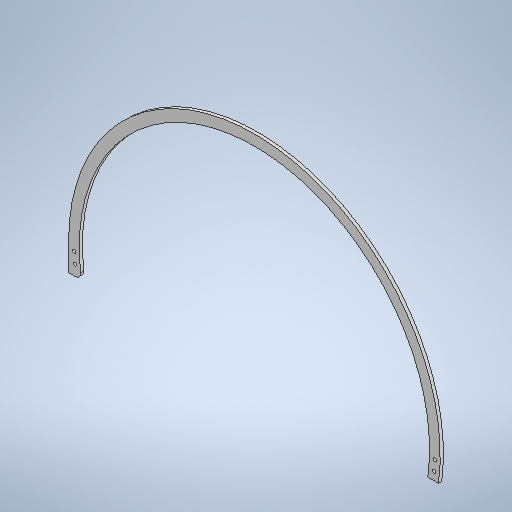
# Autodesk Inventor part: light_ball_space_out
Saved by Autodesk Inventor 2025.1 (Build 291241000, 241)
## iProperties
Created: 2025-05-06
Part Number: light_ball_space_out
Material: 一般
Document SubType Name: Modeling
Designer: yuki0520
Density: 1 g/cm^3
Appearance: 既定
Author: yuki0520
Autodesk Inventor part; units mm, degrees
ref_plane "YZ Plane" through (0, 0, 0) normal (1, 0, 0) x (0, 1, 0)
ref_plane "XZ Plane" through (0, 0, 0) normal (0, 1, 0) x (-1, 0, 0)
ref_plane "XY Plane" through (0, 0, 0) normal (0, 0, 1) x (1, 0, 0)
sketch "スケッチ1" plane through (0, 0, 0) normal (0, 0, 1) x (1, 0, 0)
  line L0 (195, -7.5) -> (-195, -7.5)
  line L1 (-195, -7.5) -> (-195, 7.5)
  line L2 (-195, 7.5) -> (195, 7.5)
  line L3 (195, 7.5) -> (195, -7.5)
  line L4 (195, -7.5) -> (-195, 7.5) construction
  line L5 (-195, -7.5) -> (195, 7.5) construction
  circle A0 centre (0, 70.8153) radius 120
  line L6 (0, -7.5) -> (0, 7.5)
  circle A1 centre (-127.5, -22.5) radius 38
  line L7 (-175, -5) -> (-135, -5)
  line L8 (-135, -5) -> (-135, 5)
  line L9 (-135, 5) -> (-175, 5)
  line L10 (-175, 5) -> (-175, -5)
  line L11 (-195, 0) -> (195, 0)
  circle A2 centre (-165, 0) radius 1.6
  circle A3 centre (-155, 0) radius 1.6
  circle A4 centre (-145, 0) radius 1.6
  line L12 (0, 190.8153) -> (0, -49.1847)
  arc A5 (156.5411, -2.2739) -> (-157.0045, 0) centre (0, 30.8153) ccw
  arc A6 (161.433, -3.3079) -> (-162.0969, 0) centre (0, 30.8153) ccw
  arc A7 (166.3249, -4.342) -> (-167.1838, 0) centre (0, 30.8153) ccw
  arc A8 (171.2168, -5.376) -> (-172.2655, 0) centre (0, 30.8153) ccw
  circle A9 centre (-169.2627, 15) radius 1.6
  circle A10 centre (-169.8998, 24.9797) radius 1.6
  line L13 (-164.9474, 34.9797) -> (-174.9504, 34.9797)
  line L14 (-175, -5) -> (-175, 30.8153)
  circle A11 centre (169.2627, 15) radius 1.6
  circle A12 centre (169.8998, 24.9797) radius 1.6
  point P0 (0, 0)
  point P1 (-145, 0)
  point P2 (-175, 0)
  point P3 (-173.0854, 5)
  point P4 (-162.968, 5)
  point P5 (163.3444, 7.5)
  point P6 (173.4399, 7.5)
  dimension "d0" = 390
  dimension "d1" = 15
  dimension "d2" = 240
  dimension "d3" = 76
  dimension "d4" = 30
  dimension "d5" = 67.5
  dimension "d9" = 10
  dimension "d10" = 10
  dimension "d11" = 30
  dimension "d13" = 10
  dimension "d14" = 10
  dimension "d16" = 3.2
  dimension "d17" = 3.2
  dimension "d19" = 3.2
  dimension "d28" = 40
  dimension "d29" = 5
  dimension "d30" = 5
  dimension "d31" = 5
  dimension "d32" = 3.2
  dimension "d33" = 3.2
  dimension "d34" = 15
  dimension "d35" = 10
  dimension "d36" = 10
  constraints: 28 end point, 15 point on circle, 13 centre point, 9 midpoint, 4 parallel, 3 coincident, 3 horizontal, 3 tangent, 3 vertical, 2 perpendicular, 2 point on line, 2 symmetric about line, 13 other
  measures "d0" distance of L1.end L2.end
  measures "d1" distance of L0.end L1.end
  measures "d2" diameter of A0
  measures "d3" diameter of A1
  measures "d4" distance from line of L2 A1.centre
  measures "d5" distance from line of L1 A1.centre
  measures "d9" distance of point (-165, 0) point (-155, 0)
  measures "d10" distance of point (-145, 0) point (-155, 0)
  measures "d11" distance from line of L1 point (-165, 0)
  measures "d13" distance of L8.end L7.end
  measures "d14" distance from line of L8 point (-145, 0)
  measures "d16" diameter of A2
  measures "d17" diameter of A3
  measures "d19" diameter of A4
  measures "d28" distance of point (0, 70.815) A5.centre
  measures "d29" radial gap between concentric circles of A5 A6
  measures "d30" radial gap between concentric circles of A6 A7
  measures "d31" radial gap between concentric circles of A7 A8
  measures "d32" diameter of A9
  measures "d33" diameter of A10
  measures "d35" distance of A10.centre A9.centre
  measures "d36" distance from line of L13 A10.centre
extrude "押し出し1" add sketch "スケッチ1" along normal blind 3 contours L2 A7 A11 A12 L13 A8 | L2 A6 L13 A7 A12 A11 | L13 A7 A10 A9 L2 A8 | A8 L2 L14 | L13 A6 L2 A7 A9 A10 | A8 L9 L14 L2 | L2 A7 L9 A8 | A6 L9 A7 L2
fillet "フィレット1" radius 5 1 edges at (-162.968, 5, 1.5)
